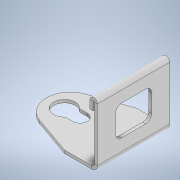
# Autodesk Inventor part: 26886-Vodička_Vojtěch-Příklad_1
Saved by Autodesk Inventor 2021 (Build 250183000, 183)
## iProperties
Created: 2022-03-21
Part Number: 26886-Vodička_Vojtěch-Příklad_1
Material: Všeobecné
Document SubType Name: Plech
Designer: 26886
Density: 1 g/cm^3
Sheet Metal Rule: Výchozí
Appearance: Výchozí
Author: 26886
Autodesk Inventor part; units mm, degrees
ref_plane "YZ Plane" through (0, 0, 0) normal (1, 0, 0) x (0, 1, 0)
ref_plane "XZ Plane" through (0, 0, 0) normal (0, 1, 0) x (-1, 0, 0)
ref_plane "XY Plane" through (0, 0, 0) normal (0, 0, 1) x (1, 0, 0)
sketch "Náčrt1" plane through (0, 0, 0) normal (0, 1, 0) x (-1, 0, 0)
  line L0 (0, 0) -> (0, -24)
  line L1 (0, -24) -> (11, -24)
  line L2 (0, 0) -> (11, 0)
  arc A0 (23.6556, -19.5464) -> (23.6556, -4.4536) centre (21, -12) ccw
  line L3 (11, 0) -> (23.6556, -4.4536)
  line L4 (11, -24) -> (23.6556, -19.5464)
  arc A1 (20.3167, -14.4) -> (20.3167, -9.6) centre (23, -12) ccw
  arc A2 (17.8, -9.6) -> (17.8, -14.4) centre (17.8, -12) ccw
  line L5 (17.8, -9.6) -> (20.3167, -9.6)
  line L6 (17.8, -14.4) -> (20.3167, -14.4)
  dimension "d0" = 24
  dimension "d1" = 11
  dimension "d3" = 16
  dimension "d4" = 7.2
  dimension "d5" = 4.8
  measures "d0" distance of L0.start L0.end
  measures "d1" distance of L0.end L1.end
  measures "d3" diameter of A0
  measures "d4" diameter of A1
  measures "d5" diameter of A2
extrude "Deska1" add sketch "Náčrt1" along normal blind 1
sketch "Náčrt2" plane through (-1, 0, -24) normal (1, 0, 0) x (0, 1, 0)
  line L0 (0, 24) -> (0, 0)
  line L1 (0, 0) -> (21, 0)
  line L2 (21, 0) -> (21, 24)
  line L3 (21, 24) -> (0, 24)
  constraints: 6 end point, 1 horizontal, 1 perpendicular, 1 vertical
edge flange "Obruba1" height 21 angle 90 thickness 1 bend radius 1 thickness toward (1, 0, 0) relief tear relief width 1 relief depth 0.5 edges at (0, 1, -12) wall of the first edge with corners at (-1, 0, 0) (-1, 0, -24) (-1, 21, -24) (-1, 21, 0)
bend "Ohyb1"
corner "Roh1"
sketch "Náčrt3" plane through (0, 21, 0) normal (1, 0, 0) x (0, 0, -1)
  line L0 (6, -13) -> (6, -7)
  line L1 (8, -5) -> (16, -5)
  line L2 (24, -19) -> (24, 0) projected
  line L3 (18, -7) -> (18, -13)
  line L4 (16, -15) -> (8, -15)
  arc A0 (8, -5) -> (6, -7) centre (8, -7) ccw
  arc A1 (18, -7) -> (16, -5) centre (16, -7) ccw
  arc A2 (16, -15) -> (18, -13) centre (16, -13) ccw
  arc A3 (6, -13) -> (8, -15) centre (8, -13) ccw
  point P0 (0, -21)
  point P1 (6, -15)
  point P2 (6, -5)
  point P3 (18, -5)
  point P4 (18, -15)
  dimension "d17" = 10
  dimension "d18" = 12
  dimension "d19" = 10
  dimension "d20" = 2
  constraints: 8 end point, 8 point on circle, 8 point on line, 8 tangent, 4 centre point, 3 equal radius, 2 perpendicular, 1 vertical
  measures "d17" distance of point (6, -15) point (6, -5)
  measures "d18" distance of point (6, -5) point (18, -5)
  measures "d19" distance of point (18, -5) point (18, -15)
  measures "d20" radius of A0
extrude "Vyříznutí1" cut sketch "Náčrt3" against normal blind 1
sketch "Náčrt4" plane through (-1, 19.75, 0) normal (0, 0, 1) x (1, 0, 0)
  line L0 (1, 0) -> (0, 0)
  arc A0 (0, 0) -> (-0.5, 0) centre (-0.25, 0) ccw
  line L1 (-0.5, 0) -> (-0.5, -2.75)
  line L2 (-0.5, -2.75) -> (-1.5, -2.75)
  line L3 (-1.5, -2.75) -> (-1.5, 0)
  arc A1 (1, 0) -> (-1.5, 0) centre (-0.25, 0) ccw
  constraints: 8 end point, 4 point on circle
hem "Lem1" sketch "Náčrt4" thickness 1 along (0, 0, -1) edges at (-1, 21, -12)
equation "\"d21\" = Tloušťka"
equation "\"d6\" = Tloušťka"
equation "\"d23\" = ŠířkaVýštipu"
equation "\"d24\" = HloubkaVýštipu"
equation "\"d25\" = MinimálníZbytek"
equation "\"d26\" = PřechodovýPoloměr"
equation "\"d27\" = 4 * Tloušťka"
equation "\"d28\" = 0.5 * Tloušťka"
equation "\"d29\" = 0.5 * d28"
equation "\"d7\" = ŠířkaVýštipu"
equation "\"d8\" = HloubkaVýštipu"
equation "\"d9\" = MinimálníZbytek"
equation "\"d10\" = PřechodovýPoloměr"
equation "\"d13\" = PoloměrOhybu"
equation "\"d14\" = VelikostRohovéhoVýštipu"
equation "\"d15\" = VelikostMezery"
equation "\"d16\" = VelikostJacobihoPoloměru"
equation "\"PoloměrOhybu\" = Tloušťka"
equation "\"ŠířkaVýštipu\" = Tloušťka"
equation "\"HloubkaVýštipu\" = 0.5 * Tloušťka"
equation "\"VelikostRohovéhoVýštipu\" = 4 * Tloušťka"
equation "\"MinimálníZbytek\" = 2 * Tloušťka"
equation "\"PřechodovýPoloměr\" = PoloměrOhybu"
equation "\"VelikostJacobihoPoloměru\" = Tloušťka"
equation "\"VelikostMezery\" = Tloušťka"
equation "\"Tloušťka\" = 1"
